Autodesk Fusion 360 part; units mm, degrees
(part 3 of 4)
  spline S621 degree 2 poles (-7.287, 4.7561) (-7.1642, 4.7561) (-7.0608, 4.7029) knots 0 0 0 1 1 1
  spline S622 degree 2 poles (-7.0608, 4.7029) (-6.9575, 4.6508) (-6.9033, 4.5597) knots 0 0 0 1 1 1
  spline S623 degree 2 poles (-6.9033, 4.5597) (-6.848, 4.4686) (-6.848, 4.3663) knots 0 0 0 1 1 1
  spline S624 degree 2 poles (-6.848, 4.3663) (-6.848, 4.2691) (-6.9002, 4.1893) knots 0 0 0 1 1 1
  spline S625 degree 2 poles (-6.9002, 4.1893) (-6.9524, 4.1095) (-7.0547, 4.0624) knots 0 0 0 1 1 1
  spline S626 degree 2 poles (-7.0547, 4.0624) (-6.9217, 4.0317) (-6.848, 3.9345) knots 0 0 0 1 1 1
  spline S627 degree 2 poles (-6.848, 3.9345) (-6.7744, 3.8383) (-6.7744, 3.693) knots 0 0 0 1 1 1
  spline S628 degree 2 poles (-6.7744, 3.693) (-6.7744, 3.4966) (-6.9176, 3.3595) knots 0 0 0 1 1 1
  spline S629 degree 2 poles (-6.9176, 3.3595) (-7.0608, 3.2234) (-7.2798, 3.2234) knots 0 0 0 1 1 1
  spline S630 degree 2 poles (-7.2798, 3.2234) (-7.4773, 3.2234) (-7.6083, 3.3411) knots 0 0 0 1 1 1
  spline S631 degree 2 poles (-7.6083, 3.3411) (-7.7382, 3.4587) (-7.7566, 3.646) knots 0 0 0 1 1 1
  line L291 (-6.5145, 3.25) -> (-6.5145, 4.75)
  line L292 (-6.5145, 4.75) -> (-5.8494, 4.75)
  spline S632 degree 2 poles (-5.8494, 4.75) (-5.6488, 4.75) (-5.5445, 4.7091) knots 0 0 0 1 1 1
  spline S633 degree 2 poles (-5.5445, 4.7091) (-5.4401, 4.6692) (-5.3777, 4.5668) knots 0 0 0 1 1 1
  spline S634 degree 2 poles (-5.3777, 4.5668) (-5.3153, 4.4645) (-5.3153, 4.3407) knots 0 0 0 1 1 1
  spline S635 degree 2 poles (-5.3153, 4.3407) (-5.3153, 4.1811) (-5.4186, 4.0716) knots 0 0 0 1 1 1
  spline S636 degree 2 poles (-5.4186, 4.0716) (-5.522, 3.9621) (-5.7379, 3.9325) knots 0 0 0 1 1 1
  spline S637 degree 2 poles (-5.7379, 3.9325) (-5.6591, 3.8946) (-5.6181, 3.8578) knots 0 0 0 1 1 1
  spline S638 degree 2 poles (-5.6181, 3.8578) (-5.5312, 3.778) (-5.4534, 3.6583) knots 0 0 0 1 1 1
  line L293 (-5.4534, 3.6583) -> (-5.1925, 3.25)
  line L294 (-5.1925, 3.25) -> (-5.4422, 3.25)
  line L295 (-5.4422, 3.25) -> (-5.6407, 3.5621)
  spline S639 degree 2 poles (-5.6407, 3.5621) (-5.7276, 3.6971) (-5.7839, 3.7688) knots 0 0 0 1 1 1
  spline S640 degree 2 poles (-5.7839, 3.7688) (-5.8402, 3.8404) (-5.8852, 3.869) knots 0 0 0 1 1 1
  spline S641 degree 2 poles (-5.8852, 3.869) (-5.9292, 3.8977) (-5.9752, 3.9089) knots 0 0 0 1 1 1
  spline S642 degree 2 poles (-5.9752, 3.9089) (-6.009, 3.9161) (-6.0857, 3.9161) knots 0 0 0 1 1 1
  line L296 (-6.0857, 3.9161) -> (-6.316, 3.9161)
  line L297 (-6.316, 3.9161) -> (-6.316, 3.25)
  line L298 (-6.316, 3.25) -> (-6.5145, 3.25)
  line L299 (-6.316, 4.088) -> (-5.8893, 4.088)
  spline S643 degree 2 poles (-5.8893, 4.088) (-5.7532, 4.088) (-5.6765, 4.1156) knots 0 0 0 1 1 1
  spline S644 degree 2 poles (-5.6765, 4.1156) (-5.5997, 4.1443) (-5.5598, 4.2057) knots 0 0 0 1 1 1
  spline S645 degree 2 poles (-5.5598, 4.2057) (-5.5199, 4.2681) (-5.5199, 4.3407) knots 0 0 0 1 1 1
  spline S646 degree 2 poles (-5.5199, 4.3407) (-5.5199, 4.4471) (-5.5977, 4.5157) knots 0 0 0 1 1 1
  spline S647 degree 2 poles (-5.5977, 4.5157) (-5.6744, 4.5842) (-5.8412, 4.5842) knots 0 0 0 1 1 1
  line L300 (-5.8412, 4.5842) -> (-6.316, 4.5842)
  line L301 (-6.316, 4.5842) -> (-6.316, 4.088)
  line L302 (-5.0063, 3.25) -> (-5.0063, 4.75)
  line L303 (-5.0063, 4.75) -> (-4.8027, 4.75)
  line L304 (-4.8027, 4.75) -> (-4.0148, 3.5723)
  line L305 (-4.0148, 3.5723) -> (-4.0148, 4.75)
  line L306 (-4.0148, 4.75) -> (-3.8245, 4.75)
  line L307 (-3.8245, 4.75) -> (-3.8245, 3.25)
  line L308 (-3.8245, 3.25) -> (-4.0281, 3.25)
  line L309 (-4.0281, 3.25) -> (-4.816, 4.4287)
  line L310 (-4.816, 4.4287) -> (-4.816, 3.25)
  line L311 (-4.816, 3.25) -> (-5.0063, 3.25)
  dimension "d71" = 4.5
  dimension "d72" = 1.5
  constraint coincident L16 L23.start
  constraint coincident L9 L23.end
  constraint perpendicular L9 L23
  constraint coincident L20 L24.start
  constraint coincident L8 L24.end
  constraint perpendicular L8 L24
  measures "d1" distance of A2.end
  measures "d71" distance of L17 L23
  measures "d72" distance of L21 L24
extrude "Extrude9" cut sketch "Sketch5" against normal blind 0.01 contours L25 S0 S1 S2 S3 S4 S5 S6 L26 S7 S8 S9 S10 S11 S12 S13 L27 S14 S15 S16 S17 S18 S19 S20 S21 S22 S23 S24 S25 S26 | L28 L29 L30 S27 S28 L31 L32 L33 S29 S30 L34 L35 L36 L37 L38 S31 S32 L39 L40 | L41 L42 L43 L44 L45 L46 | L47 L48 L49 S33 S34 L50 L51 L52 L53 L54 L55 L56 L57 L58 L59 | L60 L61 S35 S36 S37 S38 S39 S40 L62 L63 L64 | L68 S46 S47 S48 S49 S50 S51 S52 S53 S54 S55 S56 S57 S58 S59 S60 S61 S62 S63 L69 S64 S65 S66 S67 S68 S69 S70 S71 S72 S73 S74 S75 S76 S77 S78 | L70 L71 L72 S79 S80 L73 L74 L75 S81 S82 L76 L77 L78 L79 L80 S83 S84 L81 L82 | L83 S85 S86 S87 S88 S89 S90 S91 L84 S92 S93 S94 S95 S96 S97 S98 L85 S99 S100 S101 S102 S103 S104 S105 S106 S107 S108 S109 S110 S111 | S112 S113 S114 S115 S116 S117 S118 S119 S120 S121 S122 S123 | L86 L87 L88 S132 S133 L89 L90 L91 L92 | L93 L94 S134 S135 S136 S137 S138 S139 S140 S141 S142 L95 | L99 S150 S151 S152 S153 S154 S155 S156 S157 S158 S159 L100 S160 S161 S162 S163 S164 S165 S166 S167 S168 S169 | L101 L102 L103 S170 S171 L104 L105 L106 L107 | L108 L109 L110 L111 | L112 L113 S172 S173 L114 S174 S175 L115 L116 | L117 L118 S176 S177 L119 S178 S179 L120 L121 | L122 L123 L124 L125 | L126 S180 S181 S182 S183 S184 S185 S186 L127 S187 S188 S189 S190 S191 S192 S193 L128 S194 S195 S196 S197 S198 S199 S200 S201 S202 S203 S204 S205 S206 | L129 L130 S207 S208 S209 S210 S211 S212 S213 S214 S215 L131 | L135 L136 L137 L138 L139 L140 L141 L142 L143 L144 L145 | L149 L150 L151 L152 | L153 S223 S224 S225 S226 S227 S228 S229 S230 S231 S232 S233 S234 S235 S236 S237 S238 S239 S240 L154 S241 S242 S243 S244 S245 S246 S247 S248 S249 S250 S251 S252 S253 S254 S255 | L155 L156 S256 S257 S258 S259 S260 S261 S262 S263 S264 L157 | S272 S273 S274 S275 L161 S276 S277 S278 S279 L162 | L163 L164 S280 S281 L165 S282 S283 L166 L167 | L168 S284 S285 S286 S287 S288 S289 S290 S291 L169 L170 L171 L172 L173 L174 S292 S293 S294 S295 S296 S297 S298 | L175 L176 L177 S299 S300 S301 L178 S302 S303 S304 L179 | L180 S305 S306 S307 S308 L181 S309 S310 S311 S312 | S313 S314 S315 S316 S317 S318 S319 S320 S321 S322 S323 | L182 L183 S333 S334 S335 S336 S337 S338 S339 S340 S341 S342 S343 L184 | L191 S357 S358 S359 S360 S361 S362 S363 S364 S365 S366 S367 S368 S369 S370 S371 S372 S373 S374 L192 S375 S376 S377 S378 S379 S380 S381 S382 S383 S384 S385 S386 S387 S388 S389 | L193 L194 L195 L196 L197 L198 L199 L200 | L204 L205 L206 L207 | L208 L209 L210 L211 L212 L213 | L214 L215 L216 L217 L218 L219 L220 L221 L222 L223 L224 L225 | L226 S392 S393 S394 S395 S396 S397 S398 S399 S400 S401 S402 S403 S404 S405 S406 S407 S408 S409 L227 S410 S411 S412 S413 S414 S415 S416 S417 S418 S419 S420 S421 S422 S423 S424 | L228 L229 S425 S426 L230 S427 S428 L231 L232 | L233 L234 L235 L236 L237 L238 L239 L240 L241 L242 | S429 S430 S431 S432 S433 S434 S435 S436 S437 S438 S439 S440 | L243 L244 L245 L246 | L247 L248 S449 S450 L249 S451 S452 L250 L251 | L252 L253 L254 L255 L256 L257 L258 L259 | L263 S455 S456 S457 S458 S459 S460 S461 L264 S462 S463 S464 S465 S466 S467 S468 L265 S469 S470 S471 S472 S473 S474 S475 S476 S477 S478 S479 S480 S481 | S482 S483 S484 S485 S486 S487 S488 S489 S490 S491 S492 S493 | L266 L267 L268 S502 S503 L269 L270 L271 L272 | L273 L274 S504 S505 S506 S507 S508 S509 S510 S511 S512 L275 | L279 S520 S521 S522 S523 S524 S525 S526 S527 S528 S529 L280 S530 S531 S532 S533 S534 S535 S536 S537 S538 S539 | S540 S541 S542 S543 S544 S545 S546 S547 S548 S549 S550 S551 | L281 S560 S561 S562 S563 S564 S565 S566 L282 S567 S568 S569 S570 S571 S572 S573 L283 S574 S575 S576 S577 S578 S579 S580 S581 S582 S583 S584 S585 S586 | L284 L285 S587 S588 S589 S590 S591 S592 S593 S594 S595 L286 S596 S597 S598 S599 S600 S601 S602 S603 S604 L287 | L288 S605 S606 S607 S608 S609 S610 S611 L289 S612 S613 S614 S615 S616 S617 S618 L290 S619 S620 S621 S622 S623 S624 S625 S626 S627 S628 S629 S630 S631 | L291 L292 S632 S633 S634 S635 S636 S637 S638 L293 L294 L295 S639 S640 S641 S642 L296 L297 L298 | L302 L303 L304 L305 L306 L307 L308 L309 L310 L311 in component "housing"
sketch "Sketch6" plane through (0, 9, 0) normal (0, 1, 0) x (-1, 0, 0) in component "housing"
  spline S0 degree 2 poles (-6.9176, 3.3595) (-7.0608, 3.2234) (-7.2798, 3.2234) knots 0 0 0 1 1 1
  spline S1 degree 2 poles (-7.2798, 3.2234) (-7.4773, 3.2234) (-7.6083, 3.3411) knots 0 0 0 1 1 1
  spline S2 degree 2 poles (-7.6083, 3.3411) (-7.7382, 3.4587) (-7.7566, 3.646) knots 0 0 0 1 1 1
  line L0 (-7.7566, 3.646) -> (-7.5724, 3.6705)
  spline S3 degree 2 poles (-7.5724, 3.6705) (-7.5407, 3.514) (-7.465, 3.4444) knots 0 0 0 1 1 1
  spline S4 degree 2 poles (-7.465, 3.4444) (-7.3883, 3.3759) (-7.2788, 3.3759) knots 0 0 0 1 1 1
  spline S5 degree 2 poles (-7.2788, 3.3759) (-7.1488, 3.3759) (-7.0598, 3.4659) knots 0 0 0 1 1 1
  spline S6 degree 2 poles (-7.0598, 3.4659) (-6.9698, 3.5559) (-6.9698, 3.6889) knots 0 0 0 1 1 1
  spline S7 degree 2 poles (-6.9698, 3.6889) (-6.9698, 3.8158) (-7.0527, 3.8977) knots 0 0 0 1 1 1
  spline S8 degree 2 poles (-7.0527, 3.8977) (-7.1355, 3.9806) (-7.2634, 3.9806) knots 0 0 0 1 1 1
  spline S9 degree 2 poles (-7.2634, 3.9806) (-7.3156, 3.9806) (-7.3934, 3.9601) knots 0 0 0 1 1 1
  line L1 (-7.3934, 3.9601) -> (-7.3729, 4.1218)
  spline S10 degree 2 poles (-7.3729, 4.1218) (-7.3545, 4.1197) (-7.3432, 4.1197) knots 0 0 0 1 1 1
  spline S11 degree 2 poles (-7.3432, 4.1197) (-7.2256, 4.1197) (-7.1314, 4.1811) knots 0 0 0 1 1 1
  spline S12 degree 2 poles (-7.1314, 4.1811) (-7.0373, 4.2425) (-7.0373, 4.3704) knots 0 0 0 1 1 1
  spline S13 degree 2 poles (-7.0373, 4.3704) (-7.0373, 4.4717) (-7.1059, 4.5382) knots 0 0 0 1 1 1
  spline S14 degree 2 poles (-7.1059, 4.5382) (-7.1744, 4.6047) (-7.2829, 4.6047) knots 0 0 0 1 1 1
  spline S15 degree 2 poles (-7.2829, 4.6047) (-7.3903, 4.6047) (-7.4619, 4.5372) knots 0 0 0 1 1 1
  spline S16 degree 2 poles (-7.4619, 4.5372) (-7.5336, 4.4696) (-7.554, 4.3346) knots 0 0 0 1 1 1
  line L2 (-7.554, 4.3346) -> (-7.7382, 4.3673)
  spline S17 degree 2 poles (-7.7382, 4.3673) (-7.7044, 4.5525) (-7.5847, 4.6538) knots 0 0 0 1 1 1
  spline S18 degree 2 poles (-7.5847, 4.6538) (-7.465, 4.7561) (-7.287, 4.7561) knots 0 0 0 1 1 1
  spline S19 degree 2 poles (-7.287, 4.7561) (-7.1642, 4.7561) (-7.0608, 4.7029) knots 0 0 0 1 1 1
  spline S20 degree 2 poles (-7.0608, 4.7029) (-6.9575, 4.6508) (-6.9033, 4.5597) knots 0 0 0 1 1 1
  spline S21 degree 2 poles (-6.9033, 4.5597) (-6.848, 4.4686) (-6.848, 4.3663) knots 0 0 0 1 1 1
  spline S22 degree 2 poles (-6.848, 4.3663) (-6.848, 4.2691) (-6.9002, 4.1893) knots 0 0 0 1 1 1
  spline S23 degree 2 poles (-6.9002, 4.1893) (-6.9524, 4.1095) (-7.0547, 4.0624) knots 0 0 0 1 1 1
  spline S24 degree 2 poles (-7.0547, 4.0624) (-6.9217, 4.0317) (-6.848, 3.9345) knots 0 0 0 1 1 1
  spline S25 degree 2 poles (-6.848, 3.9345) (-6.7744, 3.8383) (-6.7744, 3.693) knots 0 0 0 1 1 1
  spline S26 degree 2 poles (-6.7744, 3.693) (-6.7744, 3.4966) (-6.9176, 3.3595) knots 0 0 0 1 1 1
  spline S27 degree 2 poles (11.2492, -1.6535) (11.3542, -1.9509) (11.3542, -2.2756) knots 0 0 0 1 1 1
  spline S28 degree 2 poles (11.3542, -2.2756) (11.3542, -2.6439) (11.2123, -2.9877) knots 0 0 0 1 1 1
  spline S29 degree 2 poles (11.2123, -2.9877) (11.0718, -3.3315) (10.8699, -3.588) knots 0 0 0 1 1 1
  line L3 (10.8699, -3.588) -> (10.6939, -3.588)
  spline S30 degree 2 poles (10.6939, -3.588) (11.1018, -2.9332) (11.1018, -2.2769) knots 0 0 0 1 1 1
  spline S31 degree 2 poles (11.1018, -2.2769) (11.1018, -2.0205) (11.0432, -1.7681) knots 0 0 0 1 1 1
  spline S32 degree 2 poles (11.0432, -1.7681) (10.9968, -1.5634) (10.9136, -1.3752) knots 0 0 0 1 1 1
  spline S33 degree 2 poles (10.9136, -1.3752) (10.8604, -1.2524) (10.6939, -0.9659) knots 0 0 0 1 1 1
  line L4 (10.6939, -0.9659) -> (10.8699, -0.9659)
  spline S34 degree 2 poles (10.8699, -0.9659) (11.1264, -1.3083) (11.2492, -1.6535) knots 0 0 0 1 1 1
  line L5 (3.6537, 0.9312) -> (2.4062, 0.9312)
  line L6 (2.4062, 0.9312) -> (2.4062, -0.2)
  line L7 (2.4062, -0.2) -> (2.0886, -0.2)
  line L8 (2.0886, -0.2) -> (2.0886, 2.2)
  line L9 (2.0886, 2.2) -> (2.4062, 2.2)
  line L10 (2.4062, 2.2) -> (2.4062, 1.2145)
  line L11 (2.4062, 1.2145) -> (3.6537, 1.2145)
  line L12 (3.6537, 1.2145) -> (3.6537, 2.2)
  line L13 (3.6537, 2.2) -> (3.9713, 2.2)
  line L14 (3.9713, 2.2) -> (3.9713, -0.2)
  line L15 (3.9713, -0.2) -> (3.6537, -0.2)
  line L16 (3.6537, -0.2) -> (3.6537, 0.9312)
  spline S35 degree 2 poles (4.4115, -2.8663) (4.3133, -2.9318) (4.1728, -2.9659) knots 0 0 0 1 1 1
  spline S36 degree 2 poles (4.1728, -2.9659) (4.0336, -3) (3.8522, -3) knots 0 0 0 1 1 1
  line L17 (3.8522, -3) -> (3.1305, -3)
  line L18 (3.1305, -3) -> (3.1305, -1)
  line L19 (3.1305, -1) -> (3.8194, -1)
  spline S37 degree 2 poles (3.8194, -1) (4.0527, -1) (4.1755, -1.0286) knots 0 0 0 1 1 1
  spline S38 degree 2 poles (4.1755, -1.0286) (4.3474, -1.0682) (4.4688, -1.1719) knots 0 0 0 1 1 1
  spline S39 degree 2 poles (4.4688, -1.1719) (4.6271, -1.3056) (4.7048, -1.5143) knots 0 0 0 1 1 1
  spline S40 degree 2 poles (4.7048, -1.5143) (4.784, -1.7217) (4.784, -1.9891) knots 0 0 0 1 1 1
  spline S41 degree 2 poles (4.784, -1.9891) (4.784, -2.2169) (4.7308, -2.3929) knots 0 0 0 1 1 1
  spline S42 degree 2 poles (4.7308, -2.3929) (4.6776, -2.5689) (4.5943, -2.6849) knots 0 0 0 1 1 1
  spline S43 degree 2 poles (4.5943, -2.6849) (4.5111, -2.7995) (4.4115, -2.8663) knots 0 0 0 1 1 1
  spline S44 degree 2 poles (9.4756, -2.4297) (9.5643, -2.0955) (9.7294, -1.7858) knots 0 0 0 1 1 1
  spline S45 degree 2 poles (9.7294, -1.7858) (9.8958, -1.4748) (10.0827, -1.2619) knots 0 0 0 1 1 1
  line L20 (10.0827, -1.2619) -> (9.1032, -1.2619)
  line L21 (9.1032, -1.2619) -> (9.1032, -1.0259)
  line L22 (9.1032, -1.0259) -> (10.3979, -1.0259)
  line L23 (10.3979, -1.0259) -> (10.3979, -1.2169)
  spline S46 degree 2 poles (10.3979, -1.2169) (10.2069, -1.4202) (10.0186, -1.7572) knots 0 0 0 1 1 1
  spline S47 degree 2 poles (10.0186, -1.7572) (9.8317, -2.0941) (9.7294, -2.4502) knots 0 0 0 1 1 1
  spline S48 degree 2 poles (9.7294, -2.4502) (9.6557, -2.7012) (9.6353, -3) knots 0 0 0 1 1 1
  line L24 (9.6353, -3) -> (9.3829, -3)
  spline S49 degree 2 poles (9.3829, -3) (9.387, -2.764) (9.4756, -2.4297) knots 0 0 0 1 1 1
  spline S50 degree 2 poles (8.9466, -8.8663) (8.8484, -8.9318) (8.7079, -8.9659) knots 0 0 0 1 1 1
  spline S51 degree 2 poles (8.7079, -8.9659) (8.5687, -9) (8.3873, -9) knots 0 0 0 1 1 1
  line L25 (8.3873, -9) -> (7.6656, -9)
  line L26 (7.6656, -9) -> (7.6656, -7)
  line L27 (7.6656, -7) -> (8.3545, -7)
  spline S52 degree 2 poles (8.3545, -7) (8.5878, -7) (8.7106, -7.0286) knots 0 0 0 1 1 1
  spline S53 degree 2 poles (8.7106, -7.0286) (8.8825, -7.0682) (9.0039, -7.1719) knots 0 0 0 1 1 1
  spline S54 degree 2 poles (9.0039, -7.1719) (9.1622, -7.3056) (9.2399, -7.5143) knots 0 0 0 1 1 1
  spline S55 degree 2 poles (9.2399, -7.5143) (9.3191, -7.7217) (9.3191, -7.9891) knots 0 0 0 1 1 1
  spline S56 degree 2 poles (9.3191, -7.9891) (9.3191, -8.2169) (9.2659, -8.3929) knots 0 0 0 1 1 1
  spline S57 degree 2 poles (9.2659, -8.3929) (9.2127, -8.5689) (9.1294, -8.6849) knots 0 0 0 1 1 1
  spline S58 degree 2 poles (9.1294, -8.6849) (9.0462, -8.7995) (8.9466, -8.8663) knots 0 0 0 1 1 1
  spline S59 degree 2 poles (3.7147, -5.854) (3.5237, -6.0355) (3.2318, -6.0355) knots 0 0 0 1 1 1
  spline S60 degree 2 poles (3.2318, -6.0355) (2.9685, -6.0355) (2.7938, -5.8786) knots 0 0 0 1 1 1
  spline S61 degree 2 poles (2.7938, -5.8786) (2.6206, -5.7217) (2.596, -5.472) knots 0 0 0 1 1 1
  line L28 (2.596, -5.472) -> (2.8416, -5.4393)
  spline S62 degree 2 poles (2.8416, -5.4393) (2.8839, -5.648) (2.9848, -5.7408) knots 0 0 0 1 1 1
  spline S63 degree 2 poles (2.9848, -5.7408) (3.0871, -5.8322) (3.2331, -5.8322) knots 0 0 0 1 1 1
  spline S64 degree 2 poles (3.2331, -5.8322) (3.4064, -5.8322) (3.5251, -5.7121) knots 0 0 0 1 1 1
  spline S65 degree 2 poles (3.5251, -5.7121) (3.6451, -5.5921) (3.6451, -5.4147) knots 0 0 0 1 1 1
  spline S66 degree 2 poles (3.6451, -5.4147) (3.6451, -5.2456) (3.5346, -5.1364) knots 0 0 0 1 1 1
  spline S67 degree 2 poles (3.5346, -5.1364) (3.4241, -5.0259) (3.2536, -5.0259) knots 0 0 0 1 1 1
  spline S68 degree 2 poles (3.2536, -5.0259) (3.184, -5.0259) (3.0803, -5.0532) knots 0 0 0 1 1 1
  line L29 (3.0803, -5.0532) -> (3.1076, -4.8377)
  spline S69 degree 2 poles (3.1076, -4.8377) (3.1322, -4.8404) (3.1472, -4.8404) knots 0 0 0 1 1 1
  spline S70 degree 2 poles (3.1472, -4.8404) (3.3041, -4.8404) (3.4296, -4.7585) knots 0 0 0 1 1 1
  spline S71 degree 2 poles (3.4296, -4.7585) (3.5551, -4.6767) (3.5551, -4.5061) knots 0 0 0 1 1 1
  spline S72 degree 2 poles (3.5551, -4.5061) (3.5551, -4.3711) (3.4637, -4.2824) knots 0 0 0 1 1 1
  spline S73 degree 2 poles (3.4637, -4.2824) (3.3723, -4.1937) (3.2277, -4.1937) knots 0 0 0 1 1 1
  spline S74 degree 2 poles (3.2277, -4.1937) (3.0844, -4.1937) (2.9889, -4.2838) knots 0 0 0 1 1 1
  spline S75 degree 2 poles (2.9889, -4.2838) (2.8934, -4.3738) (2.8661, -4.5539) knots 0 0 0 1 1 1
  line L30 (2.8661, -4.5539) -> (2.6206, -4.5102)
  spline S76 degree 2 poles (2.6206, -4.5102) (2.6656, -4.2633) (2.8252, -4.1282) knots 0 0 0 1 1 1
  spline S77 degree 2 poles (2.8252, -4.1282) (2.9848, -3.9918) (3.2222, -3.9918) knots 0 0 0 1 1 1
  spline S78 degree 2 poles (3.2222, -3.9918) (3.3859, -3.9918) (3.5237, -4.0628) knots 0 0 0 1 1 1
  spline S79 degree 2 poles (3.5237, -4.0628) (3.6615, -4.1323) (3.7338, -4.2538) knots 0 0 0 1 1 1
  spline S80 degree 2 poles (3.7338, -4.2538) (3.8075, -4.3752) (3.8075, -4.5116) knots 0 0 0 1 1 1
  spline S81 degree 2 poles (3.8075, -4.5116) (3.8075, -4.6412) (3.7379, -4.7476) knots 0 0 0 1 1 1
  spline S82 degree 2 poles (3.7379, -4.7476) (3.6683, -4.854) (3.5319, -4.9168) knots 0 0 0 1 1 1
  spline S83 degree 2 poles (3.5319, -4.9168) (3.7092, -4.9577) (3.8075, -5.0873) knots 0 0 0 1 1 1
  spline S84 degree 2 poles (3.8075, -5.0873) (3.9057, -5.2156) (3.9057, -5.4093) knots 0 0 0 1 1 1
  spline S85 degree 2 poles (3.9057, -5.4093) (3.9057, -5.6712) (3.7147, -5.854) knots 0 0 0 1 1 1
  line L31 (-1.5575, 0.8166) -> (-0.6522, 0.8166)
  line L32 (-0.6522, 0.8166) -> (-0.6522, 0.5203)
  line L33 (-0.6522, 0.5203) -> (-1.5575, 0.5203)
  line L34 (-1.5575, 0.5203) -> (-1.5575, 0.8166)
  spline S86 degree 2 poles (-3.7686, -2.854) (-3.9596, -3.0355) (-4.2515, -3.0355) knots 0 0 0 1 1 1
  spline S87 degree 2 poles (-4.2515, -3.0355) (-4.5148, -3.0355) (-4.6894, -2.8786) knots 0 0 0 1 1 1
  spline S88 degree 2 poles (-4.6894, -2.8786) (-4.8627, -2.7217) (-4.8872, -2.472) knots 0 0 0 1 1 1
  line L35 (-4.8872, -2.472) -> (-4.6417, -2.4393)
  spline S89 degree 2 poles (-4.6417, -2.4393) (-4.5994, -2.648) (-4.4984, -2.7408) knots 0 0 0 1 1 1
  spline S90 degree 2 poles (-4.4984, -2.7408) (-4.3961, -2.8322) (-4.2501, -2.8322) knots 0 0 0 1 1 1
  spline S91 degree 2 poles (-4.2501, -2.8322) (-4.0769, -2.8322) (-3.9582, -2.7121) knots 0 0 0 1 1 1
  spline S92 degree 2 poles (-3.9582, -2.7121) (-3.8381, -2.5921) (-3.8381, -2.4147) knots 0 0 0 1 1 1
  spline S93 degree 2 poles (-3.8381, -2.4147) (-3.8381, -2.2456) (-3.9486, -2.1364) knots 0 0 0 1 1 1
  spline S94 degree 2 poles (-3.9486, -2.1364) (-4.0591, -2.0259) (-4.2297, -2.0259) knots 0 0 0 1 1 1
  spline S95 degree 2 poles (-4.2297, -2.0259) (-4.2993, -2.0259) (-4.4029, -2.0532) knots 0 0 0 1 1 1
  line L36 (-4.4029, -2.0532) -> (-4.3756, -1.8377)
  spline S96 degree 2 poles (-4.3756, -1.8377) (-4.3511, -1.8404) (-4.3361, -1.8404) knots 0 0 0 1 1 1
  spline S97 degree 2 poles (-4.3361, -1.8404) (-4.1792, -1.8404) (-4.0537, -1.7585) knots 0 0 0 1 1 1
  spline S98 degree 2 poles (-4.0537, -1.7585) (-3.9282, -1.6767) (-3.9282, -1.5061) knots 0 0 0 1 1 1
  spline S99 degree 2 poles (-3.9282, -1.5061) (-3.9282, -1.3711) (-4.0196, -1.2824) knots 0 0 0 1 1 1
  spline S100 degree 2 poles (-4.0196, -1.2824) (-4.111, -1.1937) (-4.2556, -1.1937) knots 0 0 0 1 1 1
  spline S101 degree 2 poles (-4.2556, -1.1937) (-4.3988, -1.1937) (-4.4943, -1.2838) knots 0 0 0 1 1 1
  spline S102 degree 2 poles (-4.4943, -1.2838) (-4.5898, -1.3738) (-4.6171, -1.5539) knots 0 0 0 1 1 1
  line L37 (-4.6171, -1.5539) -> (-4.8627, -1.5102)
  spline S103 degree 2 poles (-4.8627, -1.5102) (-4.8177, -1.2633) (-4.6581, -1.1282) knots 0 0 0 1 1 1
  spline S104 degree 2 poles (-4.6581, -1.1282) (-4.4984, -0.9918) (-4.2611, -0.9918) knots 0 0 0 1 1 1
  spline S105 degree 2 poles (-4.2611, -0.9918) (-4.0973, -0.9918) (-3.9596, -1.0628) knots 0 0 0 1 1 1
  spline S106 degree 2 poles (-3.9596, -1.0628) (-3.8218, -1.1323) (-3.7495, -1.2538) knots 0 0 0 1 1 1
  spline S107 degree 2 poles (-3.7495, -1.2538) (-3.6758, -1.3752) (-3.6758, -1.5116) knots 0 0 0 1 1 1
  spline S108 degree 2 poles (-3.6758, -1.5116) (-3.6758, -1.6412) (-3.7454, -1.7476) knots 0 0 0 1 1 1
  spline S109 degree 2 poles (-3.7454, -1.7476) (-3.8149, -1.854) (-3.9514, -1.9168) knots 0 0 0 1 1 1
  spline S110 degree 2 poles (-3.9514, -1.9168) (-3.774, -1.9577) (-3.6758, -2.0873) knots 0 0 0 1 1 1
  spline S111 degree 2 poles (-3.6758, -2.0873) (-3.5776, -2.2156) (-3.5776, -2.4093) knots 0 0 0 1 1 1
  spline S112 degree 2 poles (-3.5776, -2.4093) (-3.5776, -2.6712) (-3.7686, -2.854) knots 0 0 0 1 1 1
  spline S113 degree 2 poles (-0.9129, -7.2415) (-0.9442, -7.3793) (-0.9715, -7.4761) knots 0 0 0 1 1 1
  line L38 (-0.9715, -7.4761) -> (-1.3958, -9)
  line L39 (-1.3958, -9) -> (-1.6659, -9)
  line L40 (-1.6659, -9) -> (-2.1966, -7)
  line L41 (-2.1966, -7) -> (-1.9251, -7)
  line L42 (-1.9251, -7) -> (-1.6209, -8.3111)
  spline S114 degree 2 poles (-1.6209, -8.3111) (-1.5718, -8.5171) (-1.5363, -8.7203) knots 0 0 0 1 1 1
  spline S115 degree 2 poles (-1.5363, -8.7203) (-1.4599, -8.3997) (-1.4463, -8.3506) knots 0 0 0 1 1 1
  line L43 (-1.4463, -8.3506) -> (-1.0657, -7)
  line L44 (-1.0657, -7) -> (-0.7464, -7)
  line L45 (-0.7464, -7) -> (-0.4599, -8.0123)
  spline S116 degree 2 poles (-0.4599, -8.0123) (-0.3521, -8.3888) (-0.3044, -8.7203) knots 0 0 0 1 1 1
  spline S117 degree 2 poles (-0.3044, -8.7203) (-0.2662, -8.5307) (-0.2048, -8.2851) knots 0 0 0 1 1 1
  line L46 (-0.2048, -8.2851) -> (0.109, -7)
  line L47 (0.109, -7) -> (0.375, -7)
  line L48 (0.375, -7) -> (-0.1734, -9)
  line L49 (-0.1734, -9) -> (-0.4285, -9)
  line L50 (-0.4285, -9) -> (-0.8501, -7.4761)
  spline S118 degree 2 poles (-0.8501, -7.4761) (-0.9033, -7.2851) (-0.9129, -7.2415) knots 0 0 0 1 1 1
  spline S119 degree 2 poles (-6.8245, -1.2592) (-6.6703, -1.1214) (-6.6062, -0.9918) knots 0 0 0 1 1 1
  line L51 (-6.6062, -0.9918) -> (-6.448, -0.9918)
  line L52 (-6.448, -0.9918) -> (-6.448, -3)
  line L53 (-6.448, -3) -> (-6.6935, -3)
  line L54 (-6.6935, -3) -> (-6.6935, -1.4352)
  spline S120 degree 2 poles (-6.6935, -1.4352) (-6.7822, -1.5198) (-6.9268, -1.6044) knots 0 0 0 1 1 1
  spline S121 degree 2 poles (-6.9268, -1.6044) (-7.0701, -1.6889) (-7.1847, -1.7312) knots 0 0 0 1 1 1
  line L55 (-7.1847, -1.7312) -> (-7.1847, -1.4939)
  spline S122 degree 2 poles (-7.1847, -1.4939) (-6.9787, -1.397) (-6.8245, -1.2592) knots 0 0 0 1 1 1
  spline S123 degree 2 poles (-10.6769, -0.2409) (-11.0158, -0.2409) (-11.2826, -0.0772) knots 0 0 0 1 1 1
  spline S124 degree 2 poles (-11.2826, -0.0772) (-11.5495, 0.0865) (-11.687, 0.3697) knots 0 0 0 1 1 1
  spline S125 degree 2 poles (-11.687, 0.3697) (-11.8245, 0.6529) (-11.8245, 0.9689) knots 0 0 0 1 1 1
  spline S126 degree 2 poles (-11.8245, 0.9689) (-11.8245, 1.5664) (-11.5036, 1.9037) knots 0 0 0 1 1 1
  spline S127 degree 2 poles (-11.5036, 1.9037) (-11.1827, 2.2426) (-10.6752, 2.2426) knots 0 0 0 1 1 1
  spline S128 degree 2 poles (-10.6752, 2.2426) (-10.3429, 2.2426) (-10.0761, 2.0838) knots 0 0 0 1 1 1
  spline S129 degree 2 poles (-10.0761, 2.0838) (-9.8092, 1.925) (-9.6701, 1.6401) knots 0 0 0 1 1 1
  spline S130 degree 2 poles (-9.6701, 1.6401) (-9.5293, 1.3569) (-9.5293, 0.9967) knots 0 0 0 1 1 1
  spline S131 degree 2 poles (-9.5293, 0.9967) (-9.5293, 0.6317) (-9.6766, 0.3435) knots 0 0 0 1 1 1
  spline S132 degree 2 poles (-9.6766, 0.3435) (-9.8239, 0.0554) (-10.0941, -0.0936) knots 0 0 0 1 1 1
  spline S133 degree 2 poles (-10.0941, -0.0936) (-10.3642, -0.2409) (-10.6769, -0.2409) knots 0 0 0 1 1 1
  line L56 (-11.5598, -8.764) -> (-10.5748, -8.764)
  line L57 (-10.5748, -8.764) -> (-10.5748, -9)
  line L58 (-10.5748, -9) -> (-11.8245, -9)
  line L59 (-11.8245, -9) -> (-11.8245, -7)
  line L60 (-11.8245, -7) -> (-11.5598, -7)
  line L61 (-11.5598, -7) -> (-11.5598, -8.764)
  line L62 (-9.4203, -9) -> (-9.9988, -7.2974)
  line L63 (-9.9988, -7.2974) -> (-9.9988, -9)
  line L64 (-9.9988, -9) -> (-10.2539, -9)
  line L65 (-10.2539, -9) -> (-10.2539, -7)
  line L66 (-10.2539, -7) -> (-9.8555, -7)
  line L67 (-9.8555, -7) -> (-9.3821, -8.4161)
  spline S134 degree 2 poles (-9.3821, -8.4161) (-9.3167, -8.6139) (-9.2866, -8.7121) knots 0 0 0 1 1 1
  spline S135 degree 2 poles (-9.2866, -8.7121) (-9.2525, -8.603) (-9.1802, -8.3915) knots 0 0 0 1 1 1
  line L68 (-9.1802, -8.3915) -> (-8.7014, -7)
  line L69 (-8.7014, -7) -> (-8.3453, -7)
  line L70 (-8.3453, -7) -> (-8.3453, -9)
  line L71 (-8.3453, -9) -> (-8.6004, -9)
  line L72 (-8.6004, -9) -> (-8.6004, -7.3261)
  line L73 (-8.6004, -7.3261) -> (-9.1816, -9)
  line L74 (-9.1816, -9) -> (-9.4203, -9)
  line L75 (-10.2651, -1) -> (-9.995, -1)
  line L76 (-9.995, -1) -> (-10.7781, -3)
  line L77 (-10.7781, -3) -> (-11.0496, -3)
  line L78 (-11.0496, -3) -> (-11.8245, -1)
  line L79 (-11.8245, -1) -> (-11.538, -1)
  line L80 (-11.538, -1) -> (-11.0182, -2.4529)
  spline S136 degree 2 poles (-11.0182, -2.4529) (-10.9555, -2.6276) (-10.9132, -2.7804) knots 0 0 0 1 1 1
  spline S137 degree 2 poles (-10.9132, -2.7804) (-10.8668, -2.6166) (-10.8054, -2.4529) knots 0 0 0 1 1 1
  line L81 (-10.8054, -2.4529) -> (-10.2651, -1)
  spline S138 degree 2 poles (-8.3784, -1.2592) (-8.2242, -1.1214) (-8.1601, -0.9918) knots 0 0 0 1 1 1
  line L82 (-8.1601, -0.9918) -> (-8.0018, -0.9918)
  line L83 (-8.0018, -0.9918) -> (-8.0018, -3)
  line L84 (-8.0018, -3) -> (-8.2474, -3)
  line L85 (-8.2474, -3) -> (-8.2474, -1.4352)
  spline S139 degree 2 poles (-8.2474, -1.4352) (-8.3361, -1.5198) (-8.4807, -1.6044) knots 0 0 0 1 1 1
  spline S140 degree 2 poles (-8.4807, -1.6044) (-8.6239, -1.6889) (-8.7385, -1.7312) knots 0 0 0 1 1 1
  line L86 (-8.7385, -1.7312) -> (-8.7385, -1.4939)
  spline S141 degree 2 poles (-8.7385, -1.4939) (-8.5325, -1.397) (-8.3784, -1.2592) knots 0 0 0 1 1 1
  spline S142 degree 2 poles (-2.5486, -8.854) (-2.7396, -9.0355) (-3.0315, -9.0355) knots 0 0 0 1 1 1
  spline S143 degree 2 poles (-3.0315, -9.0355) (-3.2948, -9.0355) (-3.4695, -8.8786) knots 0 0 0 1 1 1
  spline S144 degree 2 poles (-3.4695, -8.8786) (-3.6427, -8.7217) (-3.6673, -8.472) knots 0 0 0 1 1 1
  line L87 (-3.6673, -8.472) -> (-3.4217, -8.4393)
  spline S145 degree 2 poles (-3.4217, -8.4393) (-3.3794, -8.648) (-3.2785, -8.7408) knots 0 0 0 1 1 1
  spline S146 degree 2 poles (-3.2785, -8.7408) (-3.1762, -8.8322) (-3.0302, -8.8322) knots 0 0 0 1 1 1
  spline S147 degree 2 poles (-3.0302, -8.8322) (-2.8569, -8.8322) (-2.7382, -8.7121) knots 0 0 0 1 1 1
  spline S148 degree 2 poles (-2.7382, -8.7121) (-2.6182, -8.5921) (-2.6182, -8.4147) knots 0 0 0 1 1 1
  spline S149 degree 2 poles (-2.6182, -8.4147) (-2.6182, -8.2456) (-2.7287, -8.1364) knots 0 0 0 1 1 1
  spline S150 degree 2 poles (-2.7287, -8.1364) (-2.8392, -8.0259) (-3.0097, -8.0259) knots 0 0 0 1 1 1
  spline S151 degree 2 poles (-3.0097, -8.0259) (-3.0793, -8.0259) (-3.183, -8.0532) knots 0 0 0 1 1 1
  line L88 (-3.183, -8.0532) -> (-3.1557, -7.8377)
  spline S152 degree 2 poles (-3.1557, -7.8377) (-3.1311, -7.8404) (-3.1161, -7.8404) knots 0 0 0 1 1 1
  spline S153 degree 2 poles (-3.1161, -7.8404) (-2.9592, -7.8404) (-2.8337, -7.7585) knots 0 0 0 1 1 1
  spline S154 degree 2 poles (-2.8337, -7.7585) (-2.7082, -7.6767) (-2.7082, -7.5061) knots 0 0 0 1 1 1
  spline S155 degree 2 poles (-2.7082, -7.5061) (-2.7082, -7.3711) (-2.7996, -7.2824) knots 0 0 0 1 1 1
  spline S156 degree 2 poles (-2.7996, -7.2824) (-2.891, -7.1937) (-3.0356, -7.1937) knots 0 0 0 1 1 1
  spline S157 degree 2 poles (-3.0356, -7.1937) (-3.1789, -7.1937) (-3.2744, -7.2838) knots 0 0 0 1 1 1
  spline S158 degree 2 poles (-3.2744, -7.2838) (-3.3699, -7.3738) (-3.3972, -7.5539) knots 0 0 0 1 1 1
  line L89 (-3.3972, -7.5539) -> (-3.6427, -7.5102)
  spline S159 degree 2 poles (-3.6427, -7.5102) (-3.5977, -7.2633) (-3.4381, -7.1282) knots 0 0 0 1 1 1
  spline S160 degree 2 poles (-3.4381, -7.1282) (-3.2785, -6.9918) (-3.0411, -6.9918) knots 0 0 0 1 1 1
  spline S161 degree 2 poles (-3.0411, -6.9918) (-2.8774, -6.9918) (-2.7396, -7.0628) knots 0 0 0 1 1 1
  spline S162 degree 2 poles (-2.7396, -7.0628) (-2.6018, -7.1323) (-2.5295, -7.2538) knots 0 0 0 1 1 1
  spline S163 degree 2 poles (-2.5295, -7.2538) (-2.4558, -7.3752) (-2.4558, -7.5116) knots 0 0 0 1 1 1
  spline S164 degree 2 poles (-2.4558, -7.5116) (-2.4558, -7.6412) (-2.5254, -7.7476) knots 0 0 0 1 1 1
  spline S165 degree 2 poles (-2.5254, -7.7476) (-2.595, -7.854) (-2.7314, -7.9168) knots 0 0 0 1 1 1
  spline S166 degree 2 poles (-2.7314, -7.9168) (-2.5541, -7.9577) (-2.4558, -8.0873) knots 0 0 0 1 1 1
  spline S167 degree 2 poles (-2.4558, -8.0873) (-2.3576, -8.2156) (-2.3576, -8.4093) knots 0 0 0 1 1 1
  spline S168 degree 2 poles (-2.3576, -8.4093) (-2.3576, -8.6712) (-2.5486, -8.854) knots 0 0 0 1 1 1
  spline S169 degree 2 poles (-1.9541, -2.8663) (-2.0523, -2.9318) (-2.1928, -2.9659) knots 0 0 0 1 1 1
  spline S170 degree 2 poles (-2.1928, -2.9659) (-2.332, -3) (-2.5134, -3) knots 0 0 0 1 1 1
  line L90 (-2.5134, -3) -> (-3.2351, -3)
  line L91 (-3.2351, -3) -> (-3.2351, -1)
  line L92 (-3.2351, -1) -> (-2.5462, -1)
  spline S171 degree 2 poles (-2.5462, -1) (-2.3129, -1) (-2.1901, -1.0286) knots 0 0 0 1 1 1
  spline S172 degree 2 poles (-2.1901, -1.0286) (-2.0182, -1.0682) (-1.8968, -1.1719) knots 0 0 0 1 1 1
  spline S173 degree 2 poles (-1.8968, -1.1719) (-1.7385, -1.3056) (-1.6608, -1.5143) knots 0 0 0 1 1 1
  spline S174 degree 2 poles (-1.6608, -1.5143) (-1.5817, -1.7217) (-1.5817, -1.9891) knots 0 0 0 1 1 1
  spline S175 degree 2 poles (-1.5817, -1.9891) (-1.5817, -2.2169) (-1.6349, -2.3929) knots 0 0 0 1 1 1
  spline S176 degree 2 poles (-1.6349, -2.3929) (-1.6881, -2.5689) (-1.7713, -2.6849) knots 0 0 0 1 1 1
  spline S177 degree 2 poles (-1.7713, -2.6849) (-1.8545, -2.7995) (-1.9541, -2.8663) knots 0 0 0 1 1 1
  line L93 (-2.5522, 0.5269) -> (-3.5558, 0.5269)
  line L94 (-3.5558, 0.5269) -> (-3.8194, -0.2)
  line L95 (-3.8194, -0.2) -> (-4.1566, -0.2)
  line L96 (-4.1566, -0.2) -> (-3.2349, 2.2)
  line L97 (-3.2349, 2.2) -> (-2.8928, 2.2)
  line L98 (-2.8928, 2.2) -> (-1.9105, -0.2)
  line L99 (-1.9105, -0.2) -> (-2.2723, -0.2)
  line L100 (-2.2723, -0.2) -> (-2.5522, 0.5269)
  spline S178 degree 2 poles (5.1635, -5.9168) (5.0203, -6.0341) (4.8006, -6.0341) knots 0 0 0 1 1 1
  spline S179 degree 2 poles (4.8006, -6.0341) (4.5114, -6.0341) (4.3464, -5.8267) knots 0 0 0 1 1 1
  spline S180 degree 2 poles (4.3464, -5.8267) (4.1485, -5.5771) (4.1485, -5.0136) knots 0 0 0 1 1 1
  spline S181 degree 2 poles (4.1485, -5.0136) (4.1485, -4.6589) (4.2208, -4.4434) knots 0 0 0 1 1 1
  spline S182 degree 2 poles (4.2208, -4.4434) (4.2945, -4.2265) (4.4378, -4.1091) knots 0 0 0 1 1 1
  spline S183 degree 2 poles (4.4378, -4.1091) (4.5824, -3.9918) (4.8006, -3.9918) knots 0 0 0 1 1 1
  spline S184 degree 2 poles (4.8006, -3.9918) (4.9616, -3.9918) (5.083, -4.0573) knots 0 0 0 1 1 1
  spline S185 degree 2 poles (5.083, -4.0573) (5.2045, -4.1214) (5.2836, -4.2442) knots 0 0 0 1 1 1
  spline S186 degree 2 poles (5.2836, -4.2442) (5.3627, -4.3656) (5.4077, -4.5416) knots 0 0 0 1 1 1
  spline S187 degree 2 poles (5.4077, -4.5416) (5.4528, -4.7162) (5.4528, -5.0136) knots 0 0 0 1 1 1
  spline S188 degree 2 poles (5.4528, -5.0136) (5.4528, -5.3656) (5.3805, -5.5825) knots 0 0 0 1 1 1
  spline S189 degree 2 poles (5.3805, -5.5825) (5.3082, -5.7981) (5.1635, -5.9168) knots 0 0 0 1 1 1
  line L101 (7.1581, -7) -> (7.4282, -7)
  line L102 (7.4282, -7) -> (6.6451, -9)
  line L103 (6.6451, -9) -> (6.3736, -9)
  line L104 (6.3736, -9) -> (5.5987, -7)
  line L105 (5.5987, -7) -> (5.8852, -7)
  line L106 (5.8852, -7) -> (6.405, -8.4529)
  spline S190 degree 2 poles (6.405, -8.4529) (6.4678, -8.6276) (6.5101, -8.7804) knots 0 0 0 1 1 1
  spline S191 degree 2 poles (6.5101, -8.7804) (6.5564, -8.6166) (6.6178, -8.4529) knots 0 0 0 1 1 1
  line L107 (6.6178, -8.4529) -> (7.1581, -7)
  spline S192 degree 2 poles (8.9466, -5.8663) (8.8484, -5.9318) (8.7079, -5.9659) knots 0 0 0 1 1 1
  spline S193 degree 2 poles (8.7079, -5.9659) (8.5687, -6) (8.3873, -6) knots 0 0 0 1 1 1
  line L108 (8.3873, -6) -> (7.6656, -6)
  line L109 (7.6656, -6) -> (7.6656, -4)
  line L110 (7.6656, -4) -> (8.3545, -4)
  spline S194 degree 2 poles (8.3545, -4) (8.5878, -4) (8.7106, -4.0286) knots 0 0 0 1 1 1
  spline S195 degree 2 poles (8.7106, -4.0286) (8.8825, -4.0682) (9.0039, -4.1719) knots 0 0 0 1 1 1
  spline S196 degree 2 poles (9.0039, -4.1719) (9.1622, -4.3056) (9.2399, -4.5143) knots 0 0 0 1 1 1
  spline S197 degree 2 poles (9.2399, -4.5143) (9.3191, -4.7217) (9.3191, -4.9891) knots 0 0 0 1 1 1
  spline S198 degree 2 poles (9.3191, -4.9891) (9.3191, -5.2169) (9.2659, -5.3929) knots 0 0 0 1 1 1
  spline S199 degree 2 poles (9.2659, -5.3929) (9.2127, -5.5689) (9.1294, -5.6849) knots 0 0 0 1 1 1
  spline S200 degree 2 poles (9.1294, -5.6849) (9.0462, -5.7995) (8.9466, -5.8663) knots 0 0 0 1 1 1
  spline S201 degree 2 poles (5.4129, -1.764) (5.3542, -2.0191) (5.3542, -2.2769) knots 0 0 0 1 1 1
  spline S202 degree 2 poles (5.3542, -2.2769) (5.3542, -2.9332) (5.7621, -3.588) knots 0 0 0 1 1 1
  line L111 (5.7621, -3.588) -> (5.5862, -3.588)
  spline S203 degree 2 poles (5.5862, -3.588) (5.3829, -3.3315) (5.2424, -2.9877) knots 0 0 0 1 1 1
  spline S204 degree 2 poles (5.2424, -2.9877) (5.1018, -2.6439) (5.1018, -2.2756) knots 0 0 0 1 1 1
  spline S205 degree 2 poles (5.1018, -2.2756) (5.1018, -1.9509) (5.2069, -1.6535) knots 0 0 0 1 1 1
  spline S206 degree 2 poles (5.2069, -1.6535) (5.3297, -1.3083) (5.5862, -0.9659) knots 0 0 0 1 1 1
  line L112 (5.5862, -0.9659) -> (5.7621, -0.9659)
  spline S207 degree 2 poles (5.7621, -0.9659) (5.5971, -1.2497) (5.5439, -1.3711) knots 0 0 0 1 1 1
  spline S208 degree 2 poles (5.5439, -1.3711) (5.4606, -1.5593) (5.4129, -1.764) knots 0 0 0 1 1 1
  line L113 (0.2672, 0.0832) -> (1.4492, 0.0832)
  line L114 (1.4492, 0.0832) -> (1.4492, -0.2)
  line L115 (1.4492, -0.2) -> (-0.0504, -0.2)
  line L116 (-0.0504, -0.2) -> (-0.0504, 2.2)
  line L117 (-0.0504, 2.2) -> (0.2672, 2.2)
  line L118 (0.2672, 2.2) -> (0.2672, 0.0832)
  line L119 (10.8157, 0.8903) -> (9.6894, 0.8903)
  line L120 (9.6894, 0.8903) -> (9.6894, -0.2)
  line L121 (9.6894, -0.2) -> (9.3718, -0.2)
  line L122 (9.3718, -0.2) -> (9.3718, 2.2)
  line L123 (9.3718, 2.2) -> (10.9909, 2.2)
  line L124 (10.9909, 2.2) -> (10.9909, 1.9168)
  line L125 (10.9909, 1.9168) -> (9.6894, 1.9168)
  line L126 (9.6894, 1.9168) -> (9.6894, 1.1735)
  line L127 (9.6894, 1.1735) -> (10.8157, 1.1735)
  line L128 (10.8157, 1.1735) -> (10.8157, 0.8903)
  spline S209 degree 2 poles (-8.4002, 3.7156) (-8.566, 3.5764) (-8.613, 3.5263) knots 0 0 0 1 1 1
  spline S210 degree 2 poles (-8.613, 3.5263) (-8.6601, 3.4771) (-8.6908, 3.427) knots 0 0 0 1 1 1
  line L129 (-8.6908, 3.427) -> (-7.9551, 3.427)
  line L130 (-7.9551, 3.427) -> (-7.9551, 3.25)
  line L131 (-7.9551, 3.25) -> (-8.9466, 3.25)
  spline S211 degree 2 poles (-8.9466, 3.25) (-8.9486, 3.3165) (-8.9251, 3.3779) knots 0 0 0 1 1 1
  spline S212 degree 2 poles (-8.9251, 3.3779) (-8.8872, 3.4792) (-8.8044, 3.5774) knots 0 0 0 1 1 1
  spline S213 degree 2 poles (-8.8044, 3.5774) (-8.7205, 3.6756) (-8.5629, 3.8046) knots 0 0 0 1 1 1
  spline S214 degree 2 poles (-8.5629, 3.8046) (-8.3184, 4.0051) (-8.2324, 4.1218) knots 0 0 0 1 1 1
  spline S215 degree 2 poles (-8.2324, 4.1218) (-8.1465, 4.2394) (-8.1465, 4.3438) knots 0 0 0 1 1 1
  spline S216 degree 2 poles (-8.1465, 4.3438) (-8.1465, 4.4533) (-8.2252, 4.528) knots 0 0 0 1 1 1
  spline S217 degree 2 poles (-8.2252, 4.528) (-8.303, 4.6037) (-8.4289, 4.6037) knots 0 0 0 1 1 1
  spline S218 degree 2 poles (-8.4289, 4.6037) (-8.5619, 4.6037) (-8.6417, 4.5239) knots 0 0 0 1 1 1
  spline S219 degree 2 poles (-8.6417, 4.5239) (-8.7215, 4.4441) (-8.7225, 4.3029) knots 0 0 0 1 1 1
  line L132 (-8.7225, 4.3029) -> (-8.9118, 4.3223)
  spline S220 degree 2 poles (-8.9118, 4.3223) (-8.8924, 4.5341) (-8.7655, 4.6446) knots 0 0 0 1 1 1
  spline S221 degree 2 poles (-8.7655, 4.6446) (-8.6386, 4.7561) (-8.4248, 4.7561) knots 0 0 0 1 1 1
  spline S222 degree 2 poles (-8.4248, 4.7561) (-8.2089, 4.7561) (-8.083, 4.6364) knots 0 0 0 1 1 1
  spline S223 degree 2 poles (-8.083, 4.6364) (-7.9572, 4.5167) (-7.9572, 4.3397) knots 0 0 0 1 1 1
  spline S224 degree 2 poles (-7.9572, 4.3397) (-7.9572, 4.2497) (-7.994, 4.1627) knots 0 0 0 1 1 1
  spline S225 degree 2 poles (-7.994, 4.1627) (-8.0308, 4.0757) (-8.1168, 3.9795) knots 0 0 0 1 1 1
  spline S226 degree 2 poles (-8.1168, 3.9795) (-8.2017, 3.8834) (-8.4002, 3.7156) knots 0 0 0 1 1 1
  line L133 (-6.0857, 3.9161) -> (-6.316, 3.9161)
  line L134 (-6.316, 3.9161) -> (-6.316, 3.25)
  line L135 (-6.316, 3.25) -> (-6.5145, 3.25)
  line L136 (-6.5145, 3.25) -> (-6.5145, 4.75)
  line L137 (-6.5145, 4.75) -> (-5.8494, 4.75)
  spline S227 degree 2 poles (-5.8494, 4.75) (-5.6488, 4.75) (-5.5445, 4.7091) knots 0 0 0 1 1 1
  spline S228 degree 2 poles (-5.5445, 4.7091) (-5.4401, 4.6692) (-5.3777, 4.5668) knots 0 0 0 1 1 1
  spline S229 degree 2 poles (-5.3777, 4.5668) (-5.3153, 4.4645) (-5.3153, 4.3407) knots 0 0 0 1 1 1
  spline S230 degree 2 poles (-5.3153, 4.3407) (-5.3153, 4.1811) (-5.4186, 4.0716) knots 0 0 0 1 1 1
  spline S231 degree 2 poles (-5.4186, 4.0716) (-5.522, 3.9621) (-5.7379, 3.9325) knots 0 0 0 1 1 1
  spline S232 degree 2 poles (-5.7379, 3.9325) (-5.6591, 3.8946) (-5.6181, 3.8578) knots 0 0 0 1 1 1
  spline S233 degree 2 poles (-5.6181, 3.8578) (-5.5312, 3.778) (-5.4534, 3.6583) knots 0 0 0 1 1 1
  line L138 (-5.4534, 3.6583) -> (-5.1925, 3.25)
  line L139 (-5.1925, 3.25) -> (-5.4422, 3.25)
  line L140 (-5.4422, 3.25) -> (-5.6407, 3.5621)
  spline S234 degree 2 poles (-5.6407, 3.5621) (-5.7276, 3.6971) (-5.7839, 3.7688) knots 0 0 0 1 1 1
  spline S235 degree 2 poles (-5.7839, 3.7688) (-5.8402, 3.8404) (-5.8852, 3.869) knots 0 0 0 1 1 1
  spline S236 degree 2 poles (-5.8852, 3.869) (-5.9292, 3.8977) (-5.9752, 3.9089) knots 0 0 0 1 1 1
  spline S237 degree 2 poles (-5.9752, 3.9089) (-6.009, 3.9161) (-6.0857, 3.9161) knots 0 0 0 1 1 1
  spline S238 degree 2 poles (-10.4926, 3.3124) (-10.6001, 3.2244) (-10.7648, 3.2244) knots 0 0 0 1 1 1
  spline S239 degree 2 poles (-10.7648, 3.2244) (-10.9817, 3.2244) (-11.1055, 3.3799) knots 0 0 0 1 1 1
  spline S240 degree 2 poles (-11.1055, 3.3799) (-11.2539, 3.5672) (-11.2539, 3.9898) knots 0 0 0 1 1 1
  spline S241 degree 2 poles (-11.2539, 3.9898) (-11.2539, 4.2558) (-11.1997, 4.4175) knots 0 0 0 1 1 1
  spline S242 degree 2 poles (-11.1997, 4.4175) (-11.1444, 4.5802) (-11.037, 4.6681) knots 0 0 0 1 1 1
  spline S243 degree 2 poles (-11.037, 4.6681) (-10.9285, 4.7561) (-10.7648, 4.7561) knots 0 0 0 1 1 1
  spline S244 degree 2 poles (-10.7648, 4.7561) (-10.6441, 4.7561) (-10.553, 4.707) knots 0 0 0 1 1 1
  spline S245 degree 2 poles (-10.553, 4.707) (-10.4619, 4.6589) (-10.4026, 4.5668) knots 0 0 0 1 1 1
  spline S246 degree 2 poles (-10.4026, 4.5668) (-10.3432, 4.4758) (-10.3095, 4.3438) knots 0 0 0 1 1 1
  spline S247 degree 2 poles (-10.3095, 4.3438) (-10.2757, 4.2128) (-10.2757, 3.9898) knots 0 0 0 1 1 1
  spline S248 degree 2 poles (-10.2757, 3.9898) (-10.2757, 3.7258) (-10.3299, 3.5631) knots 0 0 0 1 1 1
  spline S249 degree 2 poles (-10.3299, 3.5631) (-10.3842, 3.4014) (-10.4926, 3.3124) knots 0 0 0 1 1 1
  spline S250 degree 2 poles (5.6667, -0.2409) (5.3409, -0.2409) (5.1199, -0.146) knots 0 0 0 1 1 1
  spline S251 degree 2 poles (5.1199, -0.146) (4.9005, -0.051) (4.7745, 0.1389) knots 0 0 0 1 1 1
  spline S252 degree 2 poles (4.7745, 0.1389) (4.6501, 0.3304) (4.6435, 0.5711) knots 0 0 0 1 1 1
  line L141 (4.6435, 0.5711) -> (4.9431, 0.5973)
  spline S253 degree 2 poles (4.9431, 0.5973) (4.9644, 0.4172) (5.0413, 0.301) knots 0 0 0 1 1 1
  spline S254 degree 2 poles (5.0413, 0.301) (5.1199, 0.1864) (5.2836, 0.1143) knots 0 0 0 1 1 1
  spline S255 degree 2 poles (5.2836, 0.1143) (5.4473, 0.0439) (5.652, 0.0439) knots 0 0 0 1 1 1
  spline S256 degree 2 poles (5.652, 0.0439) (5.8337, 0.0439) (5.9728, 0.098) knots 0 0 0 1 1 1
  spline S257 degree 2 poles (5.9728, 0.098) (6.112, 0.152) (6.1791, 0.2453) knots 0 0 0 1 1 1
  spline S258 degree 2 poles (6.1791, 0.2453) (6.2479, 0.3402) (6.2479, 0.4516) knots 0 0 0 1 1 1
  spline S259 degree 2 poles (6.2479, 0.4516) (6.2479, 0.5645) (6.1824, 0.648) knots 0 0 0 1 1 1
  spline S260 degree 2 poles (6.1824, 0.648) (6.1169, 0.7332) (5.9663, 0.7905) knots 0 0 0 1 1 1
  spline S261 degree 2 poles (5.9663, 0.7905) (5.8697, 0.8281) (5.539, 0.9067) knots 0 0 0 1 1 1
  spline S262 degree 2 poles (5.539, 0.9067) (5.2083, 0.9869) (5.0757, 1.0573) knots 0 0 0 1 1 1
  spline S263 degree 2 poles (5.0757, 1.0573) (4.9038, 1.1473) (4.8187, 1.2799) knots 0 0 0 1 1 1
  spline S264 degree 2 poles (4.8187, 1.2799) (4.7352, 1.4142) (4.7352, 1.5795) knots 0 0 0 1 1 1
  spline S265 degree 2 poles (4.7352, 1.5795) (4.7352, 1.7613) (4.8383, 1.9184) knots 0 0 0 1 1 1
  spline S266 degree 2 poles (4.8383, 1.9184) (4.9415, 2.0772) (5.1395, 2.1591) knots 0 0 0 1 1 1
  spline S267 degree 2 poles (5.1395, 2.1591) (5.3376, 2.2409) (5.5799, 2.2409) knots 0 0 0 1 1 1
  spline S268 degree 2 poles (5.5799, 2.2409) (5.8468, 2.2409) (6.0498, 2.1542) knots 0 0 0 1 1 1
  spline S269 degree 2 poles (6.0498, 2.1542) (6.2544, 2.069) (6.3641, 1.902) knots 0 0 0 1 1 1
  spline S270 degree 2 poles (6.3641, 1.902) (6.4738, 1.7351) (6.482, 1.5239) knots 0 0 0 1 1 1
  line L142 (6.482, 1.5239) -> (6.1775, 1.501)
  spline S271 degree 2 poles (6.1775, 1.501) (6.1529, 1.7285) (6.0105, 1.8447) knots 0 0 0 1 1 1
  spline S272 degree 2 poles (6.0105, 1.8447) (5.8697, 1.961) (5.593, 1.961) knots 0 0 0 1 1 1
  spline S273 degree 2 poles (5.593, 1.961) (5.3049, 1.961) (5.1723, 1.8546) knots 0 0 0 1 1 1
  spline S274 degree 2 poles (5.1723, 1.8546) (5.0413, 1.7498) (5.0413, 1.6008) knots 0 0 0 1 1 1
  spline S275 degree 2 poles (5.0413, 1.6008) (5.0413, 1.4715) (5.1346, 1.388) knots 0 0 0 1 1 1
  spline S276 degree 2 poles (5.1346, 1.388) (5.2263, 1.3045) (5.6127, 1.2161) knots 0 0 0 1 1 1
  spline S277 degree 2 poles (5.6127, 1.2161) (6.0007, 1.1293) (6.1447, 1.0638) knots 0 0 0 1 1 1
  spline S278 degree 2 poles (6.1447, 1.0638) (6.3543, 0.9673) (6.4541, 0.8183) knots 0 0 0 1 1 1
  spline S279 degree 2 poles (6.4541, 0.8183) (6.554, 0.6709) (6.554, 0.4778) knots 0 0 0 1 1 1
  spline S280 degree 2 poles (6.554, 0.4778) (6.554, 0.2862) (6.4443, 0.116) knots 0 0 0 1 1 1
  spline S281 degree 2 poles (6.4443, 0.116) (6.3346, -0.0527) (6.1284, -0.1476) knots 0 0 0 1 1 1
  spline S282 degree 2 poles (6.1284, -0.1476) (5.9237, -0.2409) (5.6667, -0.2409) knots 0 0 0 1 1 1
  spline S283 degree 2 poles (2.0295, -3.0341) (1.758, -3.0341) (1.5739, -2.955) knots 0 0 0 1 1 1
  spline S284 degree 2 poles (1.5739, -2.955) (1.3911, -2.8759) (1.286, -2.7176) knots 0 0 0 1 1 1
  spline S285 degree 2 poles (1.286, -2.7176) (1.1823, -2.558) (1.1769, -2.3574) knots 0 0 0 1 1 1
  line L143 (1.1769, -2.3574) -> (1.4265, -2.3356)
  spline S286 degree 2 poles (1.4265, -2.3356) (1.4443, -2.4857) (1.5084, -2.5825) knots 0 0 0 1 1 1
  spline S287 degree 2 poles (1.5084, -2.5825) (1.5739, -2.678) (1.7103, -2.7381) knots 0 0 0 1 1 1
  spline S288 degree 2 poles (1.7103, -2.7381) (1.8467, -2.7967) (2.0173, -2.7967) knots 0 0 0 1 1 1
  spline S289 degree 2 poles (2.0173, -2.7967) (2.1687, -2.7967) (2.2847, -2.7517) knots 0 0 0 1 1 1
  spline S290 degree 2 poles (2.2847, -2.7517) (2.4006, -2.7067) (2.4565, -2.6289) knots 0 0 0 1 1 1
  spline S291 degree 2 poles (2.4565, -2.6289) (2.5138, -2.5498) (2.5138, -2.457) knots 0 0 0 1 1 1
  spline S292 degree 2 poles (2.5138, -2.457) (2.5138, -2.3629) (2.4593, -2.2933) knots 0 0 0 1 1 1
  spline S293 degree 2 poles (2.4593, -2.2933) (2.4047, -2.2224) (2.2792, -2.1746) knots 0 0 0 1 1 1
  spline S294 degree 2 poles (2.2792, -2.1746) (2.1987, -2.1432) (1.9231, -2.0778) knots 0 0 0 1 1 1
  spline S295 degree 2 poles (1.9231, -2.0778) (1.6475, -2.0109) (1.537, -1.9523) knots 0 0 0 1 1 1
  spline S296 degree 2 poles (1.537, -1.9523) (1.3938, -1.8772) (1.3229, -1.7667) knots 0 0 0 1 1 1
  spline S297 degree 2 poles (1.3229, -1.7667) (1.2533, -1.6548) (1.2533, -1.5171) knots 0 0 0 1 1 1
  spline S298 degree 2 poles (1.2533, -1.5171) (1.2533, -1.3656) (1.3392, -1.2347) knots 0 0 0 1 1 1
  spline S299 degree 2 poles (1.3392, -1.2347) (1.4252, -1.1023) (1.5902, -1.0341) knots 0 0 0 1 1 1
  spline S300 degree 2 poles (1.5902, -1.0341) (1.7553, -0.9659) (1.9572, -0.9659) knots 0 0 0 1 1 1
  spline S301 degree 2 poles (1.9572, -0.9659) (2.1796, -0.9659) (2.3488, -1.0382) knots 0 0 0 1 1 1
  spline S302 degree 2 poles (2.3488, -1.0382) (2.5193, -1.1091) (2.6107, -1.2483) knots 0 0 0 1 1 1
  spline S303 degree 2 poles (2.6107, -1.2483) (2.7021, -1.3874) (2.7089, -1.5634) knots 0 0 0 1 1 1
  line L144 (2.7089, -1.5634) -> (2.4552, -1.5825)
  spline S304 degree 2 poles (2.4552, -1.5825) (2.4347, -1.3929) (2.316, -1.296) knots 0 0 0 1 1 1
  spline S305 degree 2 poles (2.316, -1.296) (2.1987, -1.1992) (1.9681, -1.1992) knots 0 0 0 1 1 1
  spline S306 degree 2 poles (1.9681, -1.1992) (1.728, -1.1992) (1.6175, -1.2879) knots 0 0 0 1 1 1
  spline S307 degree 2 poles (1.6175, -1.2879) (1.5084, -1.3752) (1.5084, -1.4993) knots 0 0 0 1 1 1
  spline S308 degree 2 poles (1.5084, -1.4993) (1.5084, -1.6071) (1.5862, -1.6767) knots 0 0 0 1 1 1
  spline S309 degree 2 poles (1.5862, -1.6767) (1.6626, -1.7462) (1.9845, -1.8199) knots 0 0 0 1 1 1
  spline S310 degree 2 poles (1.9845, -1.8199) (2.3078, -1.8922) (2.4279, -1.9468) knots 0 0 0 1 1 1
  spline S311 degree 2 poles (2.4279, -1.9468) (2.6025, -2.0273) (2.6857, -2.1514) knots 0 0 0 1 1 1
  spline S312 degree 2 poles (2.6857, -2.1514) (2.769, -2.2742) (2.769, -2.4352) knots 0 0 0 1 1 1
  spline S313 degree 2 poles (2.769, -2.4352) (2.769, -2.5948) (2.6776, -2.7367) knots 0 0 0 1 1 1
  spline S314 degree 2 poles (2.6776, -2.7367) (2.5862, -2.8772) (2.4143, -2.9563) knots 0 0 0 1 1 1
  spline S315 degree 2 poles (2.4143, -2.9563) (2.2437, -3.0341) (2.0295, -3.0341) knots 0 0 0 1 1 1
  spline S316 degree 2 poles (8.7007, -2.7913) (8.5084, -3.0341) (8.1755, -3.0341) knots 0 0 0 1 1 1
  spline S317 degree 2 poles (8.1755, -3.0341) (7.9027, -3.0341) (7.7294, -2.8813) knots 0 0 0 1 1 1
  spline S318 degree 2 poles (7.7294, -2.8813) (7.5575, -2.7285) (7.5329, -2.4761) knots 0 0 0 1 1 1
  line L145 (7.5329, -2.4761) -> (7.7908, -2.4543)
  spline S319 degree 2 poles (7.7908, -2.4543) (7.8194, -2.6426) (7.9231, -2.7381) knots 0 0 0 1 1 1
  spline S320 degree 2 poles (7.9231, -2.7381) (8.0282, -2.8322) (8.1755, -2.8322) knots 0 0 0 1 1 1
  spline S321 degree 2 poles (8.1755, -2.8322) (8.3529, -2.8322) (8.4756, -2.6985) knots 0 0 0 1 1 1
  spline S322 degree 2 poles (8.4756, -2.6985) (8.5984, -2.5648) (8.5984, -2.3438) knots 0 0 0 1 1 1
  spline S323 degree 2 poles (8.5984, -2.3438) (8.5984, -2.1337) (8.4797, -2.0123) knots 0 0 0 1 1 1
  spline S324 degree 2 poles (8.4797, -2.0123) (8.3624, -1.8909) (8.1714, -1.8909) knots 0 0 0 1 1 1
  spline S325 degree 2 poles (8.1714, -1.8909) (8.0527, -1.8909) (7.9572, -1.9454) knots 0 0 0 1 1 1
  spline S326 degree 2 poles (7.9572, -1.9454) (7.8617, -1.9986) (7.8072, -2.0846) knots 0 0 0 1 1 1
  line L146 (7.8072, -2.0846) -> (7.5766, -2.0546)
  line L147 (7.5766, -2.0546) -> (7.7703, -1.0273)
  line L148 (7.7703, -1.0273) -> (8.7649, -1.0273)
  line L149 (8.7649, -1.0273) -> (8.7649, -1.2619)
  line L150 (8.7649, -1.2619) -> (7.9668, -1.2619)
  line L151 (7.9668, -1.2619) -> (7.859, -1.7995)
  spline S327 degree 2 poles (7.859, -1.7995) (8.0391, -1.6739) (8.2369, -1.6739) knots 0 0 0 1 1 1
  spline S328 degree 2 poles (8.2369, -1.6739) (8.4988, -1.6739) (8.6789, -1.8554) knots 0 0 0 1 1 1
  spline S329 degree 2 poles (8.6789, -1.8554) (8.859, -2.0368) (8.859, -2.322) knots 0 0 0 1 1 1
  spline S330 degree 2 poles (8.859, -2.322) (8.859, -2.5935) (8.7007, -2.7913) knots 0 0 0 1 1 1
  spline S331 degree 2 poles (10.1854, -8.7135) (10.3423, -8.8076) (10.5251, -8.8076) knots 0 0 0 1 1 1
  spline S332 degree 2 poles (10.5251, -8.8076) (10.7474, -8.8076) (10.9016, -8.6794) knots 0 0 0 1 1 1
  spline S333 degree 2 poles (10.9016, -8.6794) (11.0558, -8.5512) (11.1103, -8.2988) knots 0 0 0 1 1 1
  line L152 (11.1103, -8.2988) -> (11.375, -8.3656)
  spline S334 degree 2 poles (11.375, -8.3656) (11.2918, -8.6917) (11.0749, -8.8636) knots 0 0 0 1 1 1
  spline S335 degree 2 poles (11.0749, -8.8636) (10.8593, -9.0341) (10.5469, -9.0341) knots 0 0 0 1 1 1
  spline S336 degree 2 poles (10.5469, -9.0341) (10.2236, -9.0341) (10.0203, -8.9031) knots 0 0 0 1 1 1
  spline S337 degree 2 poles (10.0203, -8.9031) (9.8184, -8.7708) (9.712, -8.5211) knots 0 0 0 1 1 1
  spline S338 degree 2 poles (9.712, -8.5211) (9.6069, -8.2715) (9.6069, -7.985) knots 0 0 0 1 1 1
  spline S339 degree 2 poles (9.6069, -7.985) (9.6069, -7.6726) (9.7256, -7.4407) knots 0 0 0 1 1 1
  spline S340 degree 2 poles (9.7256, -7.4407) (9.8457, -7.2074) (10.0653, -7.0873) knots 0 0 0 1 1 1
  spline S341 degree 2 poles (10.0653, -7.0873) (10.2863, -6.9659) (10.551, -6.9659) knots 0 0 0 1 1 1
  spline S342 degree 2 poles (10.551, -6.9659) (10.8511, -6.9659) (11.0558, -7.1187) knots 0 0 0 1 1 1